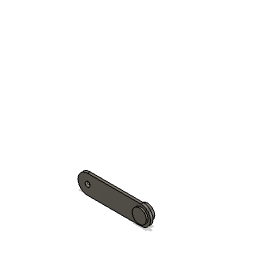
Joint 2 (Autodesk Fusion 360 design; units mm, degrees)
Autodesk Fusion 360 part; units mm, degrees
sketch "Sketch1" plane through (0, 0, 1.5) normal (0, 0, 1) x (1, 0, 0)
  circle A0 centre (356, -26.4187) radius 8.5
  circle A1 centre (356, -147.7874) radius 8.5
  arc A2 (367.5, -26.4187) -> (344.5, -26.4187) centre (356, -26.4187) ccw
  line L0 (344.5, -26.4187) -> (344.5, -147.7874)
  arc A3 (344.5, -147.7874) -> (367.5, -147.7874) centre (356, -147.7874) ccw
  line L1 (367.5, -147.7874) -> (367.5, -26.4187)
  circle A4 centre (356, -147.7874) radius 8.5
  line L2 (356, -136.2874) -> (291.8768, -136.2874)
  line L3 (356, -159.2874) -> (291.8768, -159.2874)
  arc A5 (356, -159.2874) -> (356, -136.2874) centre (356, -147.7874) ccw
  arc A6 (291.8768, -136.2874) -> (291.8768, -159.2874) centre (291.8768, -147.7874) ccw
  circle A7 centre (291.8768, -147.7874) radius 3
  dimension "d110" = 23
  dimension "d112" = 6
  constraint concentric A4 A5
  constraint tangent L2 A5
  constraint perpendicular L0 L2
  constraint midpoint A3 L3.start
  constraint tangent L3 A5
  constraint parallel L2 L3
  constraint concentric A6 A7
  measures "d110" diameter of A6
  measures "d112" diameter of A7
extrude "Extrude1" add sketch "Sketch1" along normal blind 3 contours L0 A3 L2 A5 | L0 A3 L2 L3 A6 makes body 1
extrude "Extrude1'" add sketch "Sketch1" along normal mid plane 10 separate body contours A1 A4 makes body 2 in component "Component"
component "Component" placed x (1, 0, 0) y (0, -1, 0) z (0, 0, -1) at (0, -295.5747, 3)
